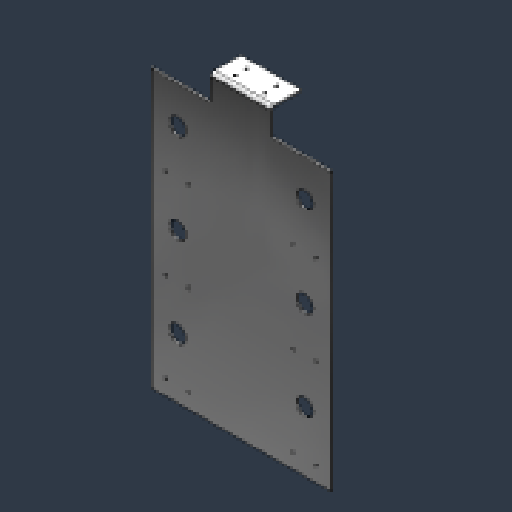
# Autodesk Inventor part: feeder_bottom_plate
Saved by Autodesk Inventor 2024.3 (Build 283343000, 343)
## iProperties
Created: 2025-03-07
Part Number: feeder_bottom_plate
Material: Aluminum 6061
Document SubType Name: Sheet Metal
Designer: marcu
Density: 2.7 g/cm^3
Sheet Metal Rule: Default
Appearance: Aluminum - Flat
Mass: 1221.59 g
Surface Area: 3039.85 cm^2
Volume: 452.44 cm^3
Author: marcu
Autodesk Inventor part; units mm, degrees
ref_plane "YZ Plane" through (0, 0, 0) normal (1, 0, 0) x (0, 1, 0)
ref_plane "XZ Plane" through (0, 0, 0) normal (0, 1, 0) x (-1, 0, 0)
ref_plane "XY Plane" through (0, 0, 0) normal (0, 0, 1) x (1, 0, 0)
sketch "Sketch1" plane through (0, 0, 0) normal (0, 0, 1) x (1, 0, 0)
  line L0 (152.4, -254) -> (-152.4, -254)
  line L1 (-152.4, -254) -> (-152.4, 254)
  line L2 (-152.4, 254) -> (152.4, 254)
  line L3 (152.4, 254) -> (152.4, -254)
  line L4 (152.4, -254) -> (-152.4, 254) construction
  line L5 (-152.4, -254) -> (152.4, 254) construction
  line L6 (-152.4, 254) -> (-50.8, 254)
  line L7 (-50.8, 254) -> (-50.8, 215.9)
  line L8 (-50.8, 215.9) -> (-152.4, 215.9)
  line L9 (-152.4, 215.9) -> (-152.4, 254)
  line L10 (152.4, 254) -> (50.8, 254)
  line L11 (50.8, 254) -> (50.8, 215.9)
  line L12 (50.8, 215.9) -> (152.4, 215.9)
  line L13 (152.4, 215.9) -> (152.4, 254)
  point P0 (0, 0)
  point P1 (-50.8, 254)
  dimension "d0" = 304.8
  dimension "d1" = 508
  dimension "d19" = 101.6
  dimension "d20" = 38.1
  dimension "d21" = 101.6
  measures "d0" distance of L1.end L2.end
  measures "d1" distance of L0.end L1.end
  measures "d19" distance of L7.end L8.end
  measures "d20" distance of L6.end L7.end
  measures "d21" distance of L12.end L11.end
extrude "Plate1" add sketch "Sketch1" along normal blind 3.048 contours L0 L1 L8 L7 L2 L11 L12 L3
sketch "Sketch2" plane through (0, 0, 0) normal (0, 0, -1) x (-1, 0, 0)
  line L0 (107.95, 152.4) -> (-107.95, 152.4) construction
  line L1 (-50.8, 254) -> (50.8, 254) construction
  line L2 (152.4, 215.9) -> (152.4, -254) construction
  point P0 (0, 0)
  point P1 (0, 152.4)
  point P2 (0, 254)
  point P3 (-152.4, 254)
  point P4 (152.4, 254)
  point P5 (107.95, 0)
  point P6 (-107.95, 0)
  point P7 (107.95, -152.4)
  point P8 (-107.95, -152.4)
  dimension "d3" = 215.9
  dimension "d4" = 101.6
  dimension "d14" = 152.4
  constraints: 2 coincident, 2 end point, 2 midpoint, 1 horizontal, 1 vertical, 1 vertical alignment, 4 other
  measures "d3" distance of L0.start L0.end
  measures "d4" distance between parallel lines of L0 L1
  measures "d14" distance of point (107.95, 152.4) point (107.95, 0)
hole "Hole1" at (-107.95, 152.4, 0) at (107.95, 152.4, 0) at (-107.95, 0, 0) at (107.95, 0, 0) at (-107.95, -152.4, 0) at (107.95, -152.4, 0) direction (0, 0, 1) diameter 28.575 end through all
sketch "Sketch3" plane through (50.8, 257.048, -3.048) normal (0, 1, 0) x (-1, 0, 0)
  line L0 (101.6, 0) -> (0, 0)
  line L1 (0, 0) -> (0, -44.704)
  line L2 (0, -44.704) -> (101.6, -44.704)
  line L3 (101.6, -44.704) -> (101.6, 0)
  constraints: 6 end point, 1 horizontal, 1 perpendicular, 1 vertical
edge flange "Flange1" height 50.8 angle 90 thickness 3.048 bend radius 3.048 thickness toward (0, 1, 0) relief straight relief width 3.048 relief depth 1.524 edges at (0, 254, 0) wall of the first edge with corners at (-50.8, 257.048, -3.048) (50.8, 257.048, -3.048) (50.8, 257.048, -47.752) (-50.8, 257.048, -47.752)
bend "Bend1"
corner "Corner1"
sketch "Sketch4" plane through (-50.8, 260.096, -47.752) normal (0, 1, 0) x (1, 0, 0)
  line L0 (126.7232, -47.752) -> (-26.9393, -47.752) construction
  line L1 (0, -44.704) -> (101.6, -44.704) construction
  line L2 (101.6, 0) -> (101.6, -44.704) construction
  line L3 (0, 0) -> (101.6, 0) construction
  line L4 (0, -44.704) -> (0, 0) construction
  point P0 (50.8, -47.752)
  point P1 (25.4, -35.052)
  point P2 (76.2, -35.052)
  point P3 (25.4, -16.002)
  point P4 (76.2, -16.002)
  dimension "d32" = 12.7
  dimension "d33" = 25.4
  dimension "d34" = 25.4
  dimension "d37" = 19.05
  constraints: 2 end point, 1 horizontal, 1 horizontal alignment, 1 vertical, 4 other
  measures "d32" distance from line of point (25.4, -35.052) L0
  measures "d33" distance from line of L4 point (25.4, -35.052)
  measures "d34" distance from line of L2 point (76.2, -35.052)
  measures "d37" distance of point (25.4, -35.052) point (25.4, -16.002)
hole "Hole2" at (-25.4, 260.096, -12.7) at (25.4, 260.096, -12.7) at (-25.4, 260.096, -31.75) at (25.4, 260.096, -31.75) direction (0, -1, 0) diameter 5.1054 end through all clearance for "Flat Head Machine Screw (82)" size "#10" standard "Ansi Unified Screw Threads"
sketch "Sketch5" plane through (0, 0, 0) normal (0, 0, -1) x (-1, 0, 0)
  circle A0 centre (-107.95, -152.4) radius 14.2875 construction
  circle A1 centre (107.95, -152.4) radius 14.2875 construction
  circle A2 centre (-107.95, 0) radius 14.2875 construction
  circle A3 centre (107.95, 0) radius 14.2875 construction
  circle A4 centre (-107.95, 152.4) radius 14.2875 construction
  circle A5 centre (107.95, 152.4) radius 14.2875 construction
  line L0 (-152.4, -254) -> (-152.4, 215.9) construction
  line L1 (152.4, -254) -> (-152.4, -254) construction
  line L2 (152.4, 215.9) -> (152.4, -254) construction
  line L3 (50.8, 215.9) -> (152.4, 215.9) construction
  line L4 (50.8, 254) -> (50.8, 215.9) construction
  line L5 (-50.8, 254) -> (50.8, 254) construction
  line L6 (-50.8, 215.9) -> (-50.8, 254) construction
  line L7 (-152.4, 215.9) -> (-50.8, 215.9) construction
  line L8 (107.95, 152.4) -> (107.95, 0) construction
  line L9 (107.95, 0) -> (107.95, -152.4) construction
  line L10 (127, 76.2) -> (88.9, 76.2) construction
  line L11 (127, -76.2) -> (88.9, -76.2) construction
  line L12 (107.95, -152.4) -> (107.95, -228.6) construction
  line L13 (127, -228.6) -> (88.9, -228.6) construction
  line L14 (0, 0) -> (0, -25.4) construction
  point P0 (107.95, 76.2)
  point P1 (107.95, -76.2)
  point P2 (-127, 76.2)
  point P3 (-88.9, 76.2)
  point P4 (-127, -76.2)
  point P5 (-88.9, -76.2)
  point P6 (-127, -228.6)
  point P7 (-88.9, -228.6)
  dimension "d49" = 38.1
  dimension "d50" = 38.1
  dimension "d51" = 76.2
  dimension "d52" = 38.1
  dimension "d53" = 25.4
  constraints: 14 end point, 6 coincident, 6 symmetric about line, 5 midpoint, 3 horizontal, 3 vertical, 1 collinear
  measures "d49" distance of L10.start L10.end
  measures "d50" distance of L11.start L11.end
  measures "d51" distance of L12.end L9.end
  measures "d52" distance of L13.start L13.end
  measures "d53" distance of L14.start L14.end
hole "Hole3" at (-127, 76.2, 0) at (-88.9, 76.2, 0) at (-127, -76.2, 0) at (-88.9, -76.2, 0) at (-127, -228.6, 0) at (-88.9, -228.6, 0) at (127, -228.6, 0) at (88.9, -228.6, 0) at (127, -76.2, 0) at (88.9, -76.2, 0) at (127, 76.2, 0) at (88.9, 76.2, 0) direction (0, 0, 1) diameter 5.1054 end through all clearance for "Flat Head Machine Screw (82)" size "#10" standard "Ansi Unified Screw Threads"
equation "\"d10\" = Thickness"
equation "\"d2\" = Thickness"
equation "\"d22\" = BendReliefWidth"
equation "\"d23\" = BendReliefDepth"
equation "\"d24\" = MinimumRemnant"
equation "\"d25\" = TransitionRadius"
equation "\"d28\" = BendRadius"
equation "\"d29\" = CornerReliefSize"
equation "\"d30\" = GapSize"
equation "\"d31\" = JacobiRadiusSize"
equation "\"d34\" = d33"
equation "\"BendRadius\" = Thickness"
equation "\"BendReliefWidth\" = Thickness"
equation "\"BendReliefDepth\" = 0.5 * Thickness"
equation "\"CornerReliefSize\" = 4 * Thickness"
equation "\"MinimumRemnant\" = 2 * Thickness"
equation "\"TransitionRadius\" = BendRadius"
equation "\"JacobiRadiusSize\" = BendRadius"
equation "\"GapSize\" = Thickness"
equation "\"Thickness\" = 3.048"
body "Solid1"
